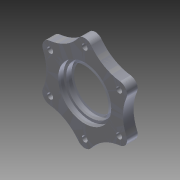
# Autodesk Inventor part: lower box bolt plate
Saved by Autodesk Inventor 2012 (Build 160160000, 160)
## iProperties
Created: 2012-12-28
Part Number: lower box bolt plate
Material: Default
Document SubType Name: Modeling
Designer: Bryce
Density: 1 g/cm^3
Translation Standard: IGES 5.3
FileName: E:\swerves\Shaft Collar.IGS
PreProcessor: SolidWorks 2012
PostProcessor: Build: 160, Release: 2012 RTM - Date: Tue 03/01/2011
Sent Units: inch
Uncertainty: 1e-08
Author: Bryce
Autodesk Inventor part; units mm, degrees
ref_plane "YZ Plane" through (0, 0, 0) normal (1, 0, 0) x (0, 1, 0)
ref_plane "XZ Plane" through (0, 0, 0) normal (0, 1, 0) x (-1, 0, 0)
ref_plane "XY Plane" through (0, 0, 0) normal (0, 0, 1) x (1, 0, 0)
surface "Composite1"
sketch "Sketch2" plane through (0, -23.8125, 0) normal (0, 0, 1) x (1, 0, 0)
  arc A0 (3.8159, 50.4746) -> (21.182, 40.4482) centre (24.1677, 65.6722) ccw projected
  arc A1 (3.8159, 50.4746) -> (-3.8159, 50.4746) centre (0, 47.625) ccw projected
  arc A2 (-21.182, 40.4482) -> (-3.8159, 50.4746) centre (-24.1677, 65.6722) ccw projected
  arc A3 (-21.182, 40.4482) -> (-24.998, 33.8388) centre (-20.6222, 35.7187) ccw projected
  arc A4 (-24.998, 13.7862) -> (-24.998, 33.8388) centre (-48.3354, 23.8125) ccw projected
  arc A5 (-24.998, 13.7862) -> (-21.182, 7.1768) centre (-20.6222, 11.9062) ccw projected
  arc A6 (-3.8159, -2.8496) -> (-21.182, 7.1768) centre (-24.1677, -18.0472) ccw projected
  arc A7 (-3.8159, -2.8496) -> (3.8159, -2.8496) centre (0, 0) ccw projected
  arc A8 (21.182, 7.1768) -> (3.8159, -2.8496) centre (24.1677, -18.0472) ccw projected
  arc A9 (21.182, 7.1768) -> (24.998, 13.7862) centre (20.6222, 11.9063) ccw projected
  arc A10 (24.998, 33.8388) -> (24.998, 13.7862) centre (48.3354, 23.8125) ccw projected
  arc A11 (24.998, 33.8388) -> (21.182, 40.4482) centre (20.6222, 35.7188) ccw projected
  circle A12 centre (0, 47.625) radius 1.7272 projected
  circle A13 centre (20.6222, 35.7188) radius 1.7272 projected
  circle A14 centre (20.6222, 11.9063) radius 1.7272 projected
  circle A15 centre (0, 0) radius 1.7272 projected
  circle A16 centre (-20.6222, 11.9062) radius 1.7272 projected
  circle A17 centre (-20.6222, 35.7187) radius 1.7272 projected
  arc A18 (14.2875, 23.8125) -> (-14.2875, 23.8125) centre (0, 23.8125) ccw projected
  arc A19 (-14.2875, 23.8125) -> (14.2875, 23.8125) centre (0, 23.8125) ccw projected
  circle A20 centre (0, 23.8125) radius 12.7 projected
extrude "Extrusion1" add sketch "Sketch2" along normal blind 6.35 contours A0 A11 A10 A9 A8 A7 A6 A5 A4 A3 A2 A1
extrude "Extrusion2" add sketch "Sketch2" along normal blind 3.175 contours A19 A18
sketch "Sketch3" plane through (0, -23.8125, 6.35) normal (0, 0, 1) x (1, 0, 0)
  circle A0 centre (0, 23.8125) radius 14.2875 projected
  circle A1 centre (0, 23.8125) radius 15.875
  circle A2 centre (0, 23.8125) radius 12.7 projected
  dimension "d4" = 31.75
  constraints: 1 centre point, 1 coincident
  measures "d4" diameter of A1
extrude "Extrusion3" cut sketch "Sketch3" against normal blind 3.175 contours A1
extrude "Extrusion4" cut sketch "Sketch3" against normal through all contours A0
chamfer "Chamfer1" distance 2.9972 angle 45 6 edges at (18.895, 11.9063, 0) (-1.7272, 23.8125, 0) (-22.3494, 11.9063, 0) (-22.3494, -11.9062, 0) (-1.7272, -23.8125, 0) (18.895, -11.9062, 0)
body "Solid1"
body "Srf1"
